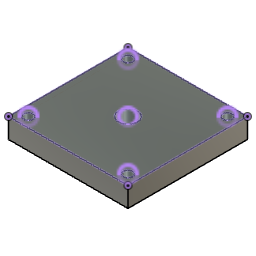
topcap v3 (Autodesk Fusion 360 design; units mm, degrees)
Autodesk Fusion 360 part; units mm, degrees
sketch "Sketch1" plane through (0, 0, 0) normal (0, 0, 1) x (1, 0, 0)
  line L0 (38.1, -38.1) -> (-38.1, -38.1)
  line L1 (-38.1, -38.1) -> (-38.1, 38.1)
  line L2 (-38.1, 38.1) -> (38.1, 38.1)
  line L3 (38.1, 38.1) -> (38.1, -38.1)
  line L4 (38.1, -38.1) -> (-38.1, 38.1) construction
  line L5 (-38.1, -38.1) -> (38.1, 38.1) construction
  line L6 (31.75, 31.75) -> (-31.75, 31.75) construction
  line L7 (-31.75, 31.75) -> (-31.75, -31.75) construction
  line L8 (-31.75, -31.75) -> (31.75, -31.75) construction
  line L9 (31.75, -31.75) -> (31.75, 31.75) construction
  line L10 (31.75, 31.75) -> (-31.75, -31.75) construction
  line L11 (-31.75, 31.75) -> (31.75, -31.75) construction
  circle A0 centre (-31.75, 31.75) radius 3
  circle A1 centre (-31.75, -31.75) radius 3
  circle A2 centre (31.75, -31.75) radius 3
  circle A3 centre (31.75, 31.75) radius 3
  circle A4 centre (0, 0) radius 6
  dimension "d1" = 76.2
  dimension "d2" = 76.2
  dimension "d3" = 63.5
  dimension "d4" = 63.5
  dimension "d5" = 6
  dimension "d7" = 360
  dimension "d10" = 12
  constraint horizontal L0
  constraint perpendicular L0 L1
  constraint parallel L0 L2
  constraint parallel L1 L3
  constraint coincident L4 A4.centre
  constraint coincident L5 A4.centre
  constraint coincident A4.centre origin
  constraint horizontal L6
  constraint perpendicular L6 L7
  constraint parallel L6 L8
  constraint parallel L7 L9
  constraint coincident L10 A4.centre
  constraint coincident L11 A4.centre
  constraint coincident L6.end L7.start
  measures "d1" distance of L1.end L2.end
  measures "d2" distance of L0.end L1.end
  measures "d3" distance of L7.end L8.end
  measures "d4" distance of L6.end L7.end
  measures "d5" diameter of A0
  measures "d10" diameter of A4
extrude "Extrude1" add sketch "Sketch1" along normal blind 12.7
sketch "Sketch2" plane through (0, 0, 12.7) normal (0, 0, 1) x (-1, 0, 0)
  circle A0 centre (31.75, -31.75) radius 3
  circle A1 centre (0, 0) radius 6
  circle A2 centre (31.75, 31.75) radius 3
  circle A3 centre (-31.75, -31.75) radius 3
  circle A4 centre (-31.75, 31.75) radius 3
  line L0 (-38.1, -38.1) -> (38.1, -38.1)
  line L1 (38.1, -38.1) -> (38.1, 38.1)
  line L2 (38.1, 38.1) -> (-38.1, 38.1)
  line L3 (-38.1, 38.1) -> (-38.1, -38.1)
